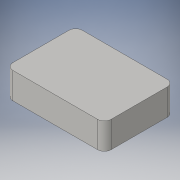
# Autodesk Inventor part: Case
Saved by Autodesk Inventor 2016 (Build 200138000, 138)
## iProperties
Created: 2016-03-01
Part Number: Case
Material: Generic
Document SubType Name: Modeling
Designer: agmle
Density: 1 g/cm^3
Appearance: Default
Author: agmle
Autodesk Inventor part; units mm, degrees
ref_plane "YZ Plane" through (0, 0, 0) normal (1, 0, 0) x (0, 1, 0)
ref_plane "XZ Plane" through (0, 0, 0) normal (0, 1, 0) x (-1, 0, 0)
ref_plane "XY Plane" through (0, 0, 0) normal (0, 0, 1) x (1, 0, 0)
sketch "Sketch1" plane through (0, 0, 0) normal (0, 1, 0) x (-1, 0, 0)
  line L0 (161.1, 132) -> (-161.1, 132)
  line L1 (-186.5, 106.6) -> (-186.5, -106.6)
  line L2 (-161.1, -132) -> (161.1, -132)
  line L3 (186.5, -106.6) -> (186.5, 106.6)
  line L4 (0, -132) -> (0, 132) construction
  arc A0 (161.1, -132) -> (186.5, -106.6) centre (161.1, -106.6) ccw
  arc A1 (-186.5, -106.6) -> (-161.1, -132) centre (-161.1, -106.6) ccw
  arc A2 (-161.1, 132) -> (-186.5, 106.6) centre (-161.1, 106.6) ccw
  arc A3 (186.5, 106.6) -> (161.1, 132) centre (161.1, 106.6) ccw
  point P0 (0, 0)
  point P1 (186.5, 132)
  point P2 (-186.5, -132)
  point P3 (186.5, -132)
  point P4 (0, 0)
  dimension "d0" = 264
  dimension "d1" = 373
  dimension "d2" = 25.4
  constraints: 10 end point, 8 point on circle, 8 tangent, 6 point on line, 4 centre point, 3 equal radius, 3 midpoint, 2 parallel, 1 coincident, 1 horizontal, 1 perpendicular
  measures "d0" distance of point (186.5, -132) point (186.5, 132)
  measures "d1" distance of point (-186.5, -132) point (186.5, -132)
  measures "d2" radius of A0
extrude "Extrusion1" add sketch "Sketch1" along normal blind 100
body "Solid1"
